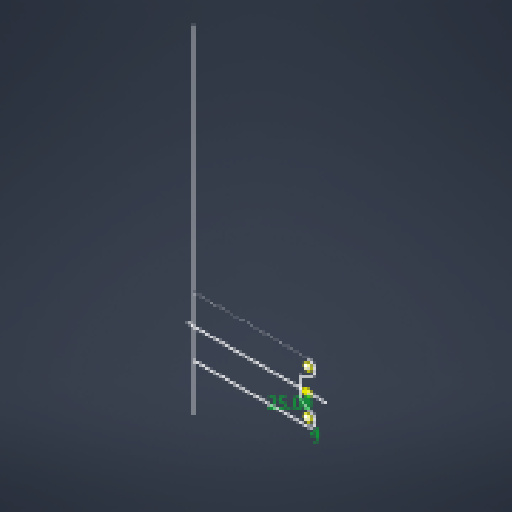
# Autodesk Inventor part: Motordriver_Adapter
Saved by Autodesk Inventor 2023.4 (Build 274418000, 418)
## iProperties
Created: 2025-10-22
Part Number: Motordriver_Adapter
Material: Generic
Document SubType Name: Modeling
Designer: Malthe Sennels
Density: 1 g/cm^3
Appearance: Default
Author: Malthe Sennels
Autodesk Inventor part; units mm, degrees
ref_plane "YZ Plane" through (0, 0, 0) normal (1, 0, 0) x (0, 1, 0)
ref_plane "XZ Plane" through (0, 0, 0) normal (0, 1, 0) x (-1, 0, 0)
ref_plane "XY Plane" through (0, 0, 0) normal (0, 0, 1) x (1, 0, 0)
sketch "Sketch1" plane through (0, 0, 0) normal (0, 0, 1) x (1, 0, 0)
  circle A0 centre (1.5276, -12) radius 1.75
  circle A1 centre (1.5276, 0) radius 1.75
  circle A2 centre (1.5276, 12) radius 1.75
  arc A3 (1.5276, -16) -> (3.2181, -8.3748) centre (1.5276, -12) ccw
  line L0 (3.2181, -8.3748) -> (-2.4724, -5.7213)
  line L1 (1.5276, -16) -> (-60.6, -16)
  line L2 (11.3984, 0) -> (-64.1078, 0)
  line L3 (-60.6, 141.7) -> (-60.6, -41.7)
  line L4 (-2.4724, -5.7213) -> (-2.4724, 0)
  arc A4 (3.2181, 8.3748) -> (1.5276, 16) centre (1.5276, 12) ccw
  line L5 (3.2181, 8.3748) -> (-2.4724, 5.7213)
  line L6 (1.5276, 16) -> (-60.6, 16) construction
  line L7 (-2.4724, 5.7213) -> (-2.4724, 0)
  circle A5 centre (-32.0875, 25.9484) radius 1.6
  circle A6 centre (-44.5875, -20.9516) radius 1.6
  circle A7 centre (-109.5875, -20.9516) radius 1.6
  circle A8 centre (-109.5875, 17.8984) radius 1.6
  line L8 (-30.6, -16) -> (-40.6, -26)
  line L9 (-30.6, -16) -> (-16.4579, -16) construction
  line L10 (-40.6, -26) -> (-60.6, -26)
  line L11 (1.5276, 16) -> (-23.224, 16)
  line L12 (-23.224, 16) -> (-31.224, 24) construction
  line L13 (-23.224, 16) -> (-11.9103, 16) construction
  line L14 (-31.224, 24) -> (-109.7276, 24)
  line L15 (-109.7276, 24) -> (-117.7276, 16)
  circle A9 centre (-122.7276, -12) radius 1.75
  circle A10 centre (-122.7276, 0) radius 1.75
  circle A11 centre (-122.7276, 12) radius 1.75
  arc A12 (-124.4181, -8.3748) -> (-122.7276, -16) centre (-122.7276, -12) ccw
  arc A13 (-122.7276, 16) -> (-124.4181, 8.3748) centre (-122.7276, 12) ccw
  line L16 (-122.7276, 16) -> (-117.7276, 16)
  line L17 (-60.6, -26) -> (-112.7276, -26)
  line L18 (-112.7276, -26) -> (-122.7276, -16)
  line L19 (-124.4181, -8.3748) -> (-118.7276, -5.7213)
  line L20 (-118.7276, -5.7213) -> (-118.7276, 0)
  line L21 (-118.7276, 5.7213) -> (-118.7276, 0)
  line L22 (-124.4181, 8.3748) -> (-118.7276, 5.7213)
  line L23 (-11.9103, 16) -> (-25.5298, 29.6196)
  line L24 (-11.9103, 16) -> (7.3507, 16) construction
  line L25 (-25.5298, 29.6196) -> (-40.2322, 29.6196)
  line L26 (-40.2322, 29.6196) -> (-45.8517, 24)
  line L27 (-12.954, -10.4954) -> (-41.3116, -10.4954)
  line L28 (-41.3116, -10.4954) -> (-50.8162, -20)
  line L29 (-50.8162, -20) -> (-99.9221, -20)
  line L30 (-99.9221, -20) -> (-110.7276, -9.1945)
  line L31 (-110.7276, -9.1945) -> (-110.7276, 3.4171)
  line L32 (-110.7276, 3.4171) -> (-98.1447, 16)
  line L33 (-98.1447, 16) -> (-21.5239, 16)
  line L34 (-21.5239, 16) -> (-17.2785, 11.7546)
  line L35 (-17.2785, 11.7546) -> (-17.448, 11.7546)
  line L36 (-17.448, 11.7546) -> (-8.8369, 3.1435)
  line L37 (-8.8369, 3.1435) -> (-8.8369, -6.3783)
  line L38 (-8.8369, -6.3783) -> (-12.954, -10.4954)
  point P0 (0, 0)
extrude "Extrusion1" add sketch "Sketch1" along normal blind 3 contours L4 L0 A3 L1 L28 L27 L38 L37 L2 | L2 L37 L36 L35 L34 L11 A4 L5 L7 | L33 L32 L31 L30 L29 L3 L17 L18 A12 L19 L20 L21 L22 A13 L16 L15 L14 | L3 L14 L26 L25 L23 L11 L33 | L1 L8 L10 L3 L29 L28
sketch "Sketch2" plane through (0, 0, 3) normal (0, 0, 1) x (1, 0, 0)
  circle A0 centre (-32.0875, 25.9484) radius 1.6 projected
  circle A1 centre (-44.5875, -20.9516) radius 1.6 projected
  circle A2 centre (-109.5875, -20.9516) radius 1.6 projected
  circle A3 centre (-109.5875, 17.8984) radius 1.6 projected
  circle A4 centre (-109.5875, -20.9516) radius 3.25
  circle A5 centre (-109.5875, 17.8984) radius 3.25
  circle A6 centre (-32.0875, 25.9484) radius 3.25
  circle A7 centre (-44.5875, -20.9516) radius 1.6 projected
  circle A8 centre (-44.5875, -20.9516) radius 3.25
  point P0 (0, 0)
  dimension "d15" = 6.5
  dimension "d16" = 6.5
  dimension "d17" = 6.5
  dimension "d18" = 6.5
  constraints: 4 centre point, 4 coincident
  measures "d15" diameter of A4
  measures "d16" diameter of A5
  measures "d17" diameter of A6
  measures "d18" diameter of A8
extrude "Extrusion2" add sketch "Sketch2" along normal blind 4
body "Solid1"
